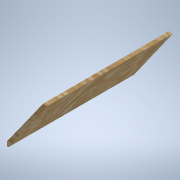
# Autodesk Inventor part: Backplane
Saved by Autodesk Inventor 2021 (Build 250183000, 183)
## iProperties
Created: 2020-07-16
Part Number: Backplane
Material: Generic
Document SubType Name: Modeling
Designer: adick
Density: 1 g/cm^3
Appearance: Plywood - Weathered
Author: adick
Autodesk Inventor part; units mm, degrees
ref_plane "YZ Plane" through (0, 0, 0) normal (1, 0, 0) x (0, 1, 0)
ref_plane "XZ Plane" through (0, 0, 0) normal (0, 1, 0) x (-1, 0, 0)
ref_plane "XY Plane" through (0, 0, 0) normal (0, 0, 1) x (1, 0, 0)
sketch "Sketch1" plane through (0, 0, 0) normal (0, 0, 1) x (1, 0, 0)
  line L0 (67.8086, 112.822) -> (-59.1914, -66.8193) projected
  line L1 (-69.85, 119.8) -> (69.85, 119.8) projected
  line L2 (67.8086, 119.8) -> (-65.0875, -68.2625)
  line L3 (-69.85, -61.8748) -> (-69.85, -68.2625)
  line L4 (-69.85, -68.2625) -> (-65.0875, -68.2625)
  line L5 (67.8086, 119.8) -> (53.3144, 119.8)
  line L6 (53.3144, 119.8) -> (-69.85, -52.9916)
  line L7 (-69.85, -52.9916) -> (-69.85, -61.8748)
  point P0 (0, 0)
  constraints: 12 end point, 2 vertical, 1 collinear, 1 perpendicular, 1 point on line
extrude "Extrusion1" add sketch "Sketch1" along normal blind 430
body "Solid1"
